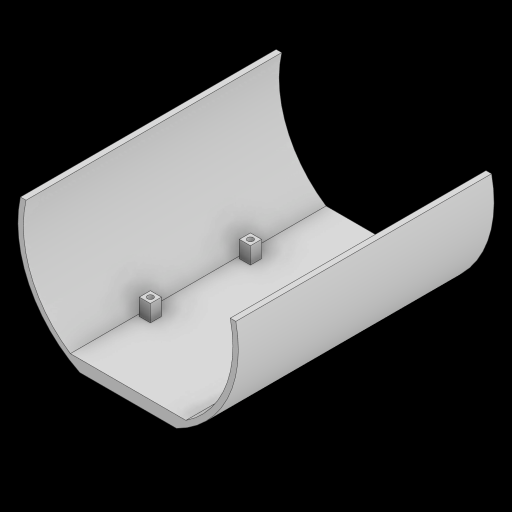
# Autodesk Inventor part: BackInsertV1
Saved by Autodesk Inventor 2024 (Build 280153000, 153)
## iProperties
Created: 2026-04-20
Part Number: BackInsertV1
Material: Generic
Document SubType Name: Modeling
Designer: Tanner
Density: 1 g/cm^3
Appearance: Default
Author: Tanner
## iProperties of the stored document BackInsertV1_3DPrint.ipt
Created: 2026-04-27
Part Number: BackInsertV1_3DPrint
Material: Generic
Document SubType Name: Modeling
Designer: Tanner
Density: 1 g/cm^3
Appearance: Default
Author: Tanner
Autodesk Inventor part; units mm, degrees
ref_plane "YZ Plane" through (0, 0, 0) normal (1, 0, 0) x (0, 1, 0)
ref_plane "XZ Plane" through (0, 0, 0) normal (0, 1, 0) x (-1, 0, 0)
ref_plane "XY Plane" through (0, 0, 0) normal (0, 0, 1) x (1, 0, 0)
sketch "Sketch1" plane through (0, 0, 0) normal (0, 0, 1) x (1, 0, 0)
  arc A0 (-96.8589, 55) -> (-43.4971, -55) centre (0, 34.0439) ccw projected
  line L0 (-43.4971, -55) -> (43.4971, -55) projected
  arc A1 (43.4971, -55) -> (96.8589, 55) centre (0, 34.0439) ccw projected
  line L1 (96.8589, 55) -> (91.8589, 55) projected
  arc A2 (51.9882, -44.5338) -> (91.8589, 55) centre (0, 34.0439) ccw projected
  arc A3 (-91.8589, 55) -> (-51.9882, -44.5338) centre (0, 34.0439) ccw projected
  line L2 (-91.8589, 55) -> (-96.8589, 55) projected
  line L3 (51.9882, -44.5338) -> (-51.9882, -44.5338) projected
  point P0 (0, 0)
extrude "Extrusion1" add sketch "Sketch1" along normal blind 230
sketch "Sketch2" plane through (-43.4971, -44.5338, 0) normal (0, 1, 0) x (1, 0, 0)
  circle A0 centre (-1.5029, -75) radius 1.6 construction
  circle A1 centre (-1.5029, -165) radius 1.6 construction
  circle A2 centre (88.4971, -75) radius 1.6 construction
  circle A3 centre (88.4971, -165) radius 1.6 construction
  line L0 (-6.5029, -70) -> (-6.5029, -170) construction
  line L1 (-6.5029, -170) -> (93.4971, -170) construction
  line L2 (93.4971, -170) -> (93.4971, -70) construction
  line L3 (93.4971, -70) -> (-6.5029, -70) construction
  line L4 (86.9943, 0) -> (0, 0) construction
  line L5 (0, 0) -> (0, -230) construction
  line L6 (86.9943, -230) -> (0, -230) construction
  line L7 (86.9943, 0) -> (86.9943, -230) construction
  line L8 (-6.5029, -80) -> (3.4971, -80)
  line L9 (3.4971, -80) -> (3.4971, -70)
  line L10 (3.4971, -70) -> (-6.5029, -70)
  line L11 (-6.5029, -70) -> (-6.5029, -80)
  line L12 (-6.5029, -80) -> (3.4971, -70) construction
  line L13 (3.4971, -80) -> (-6.5029, -70) construction
  line L14 (83.4971, -80) -> (93.4971, -80)
  line L15 (93.4971, -80) -> (93.4971, -70)
  line L16 (93.4971, -70) -> (83.4971, -70)
  line L17 (83.4971, -70) -> (83.4971, -80)
  line L18 (83.4971, -80) -> (93.4971, -70) construction
  line L19 (93.4971, -80) -> (83.4971, -70) construction
  line L20 (3.4971, -170) -> (-6.5029, -170)
  line L21 (-6.5029, -170) -> (-6.5029, -160)
  line L22 (-6.5029, -160) -> (3.4971, -160)
  line L23 (3.4971, -160) -> (3.4971, -170)
  line L24 (3.4971, -170) -> (-6.5029, -160) construction
  line L25 (-6.5029, -170) -> (3.4971, -160) construction
  line L26 (83.4971, -170) -> (93.4971, -170)
  line L27 (93.4971, -170) -> (93.4971, -160)
  line L28 (93.4971, -160) -> (83.4971, -160)
  line L29 (83.4971, -160) -> (83.4971, -170)
  line L30 (83.4971, -170) -> (93.4971, -160) construction
  line L31 (93.4971, -170) -> (83.4971, -160) construction
  point P0 (43.4971, 0)
  dimension "d2" = 10
  dimension "d3" = 10
  dimension "d4" = 10
  dimension "d5" = 10
  dimension "d6" = 10
  dimension "d7" = 10
  dimension "d8" = 10
  dimension "d9" = 10
  constraints: 48 end point, 8 midpoint, 8 parallel, 4 horizontal, 4 perpendicular
  measures "d2" distance of L10.end L9.end
  measures "d3" distance of L9.end L8.end
  measures "d4" distance of L16.end L15.end
  measures "d5" distance of L15.end L14.end
  measures "d6" distance of L21.end L22.end
  measures "d7" distance of L20.end L21.end
  measures "d8" distance of L28.end L27.end
  measures "d9" distance of L27.end L26.end
extrude "Extrusion2" add sketch "Sketch2" along normal blind 15
sketch "Sketch3" plane through (-43.4971, -29.5338, 0) normal (0, 1, 0) x (1, 0, 0)
  circle A0 centre (-1.5029, -75) radius 1.6 construction
  circle A1 centre (-1.5029, -165) radius 1.6 construction
  circle A2 centre (88.4971, -75) radius 1.6 construction
  circle A3 centre (88.4971, -165) radius 1.6 construction
  line L0 (-6.5029, -70) -> (-6.5029, -170) construction
  line L1 (-6.5029, -170) -> (93.4971, -170) construction
  line L2 (93.4971, -170) -> (93.4971, -70) construction
  line L3 (93.4971, -70) -> (-6.5029, -70) construction
  circle A4 centre (-1.5029, -75) radius 2.665
  circle A5 centre (88.4971, -75) radius 2.665
  circle A6 centre (88.4971, -165) radius 2.665
  circle A7 centre (-1.5029, -165) radius 2.665
  point P0 (43.4971, 0)
  dimension "d12" = 5.33
  dimension "d13" = 5.33
  dimension "d14" = 5.33
  dimension "d15" = 5.33
  constraints: 4 centre point, 4 coincident
  measures "d12" diameter of A4
  measures "d13" diameter of A5
  measures "d14" diameter of A6
  measures "d15" diameter of A7
extrude "Extrusion3" cut sketch "Sketch3" against normal blind 11.5
sketch "Sketch4" plane through (0, 0, 0) normal (0, 0, -1) x (-1, 0, 0)
  arc A0 (43.4971, -55) -> (96.8589, 55) centre (0, 34.0439) ccw construction
  line L0 (43.4971, -55) -> (-43.4971, -55) construction
  arc A1 (-96.8589, 55) -> (-43.4971, -55) centre (0, 34.0439) ccw construction
  line L1 (-96.8589, 55) -> (-91.8589, 55) construction
  arc A2 (-91.8589, 55) -> (-51.9882, -44.5338) centre (0, 34.0439) ccw construction
  line L2 (-51.9882, -44.5338) -> (51.9882, -44.5338) construction
  arc A3 (51.9882, -44.5338) -> (91.8589, 55) centre (0, 34.0439) ccw construction
  line L3 (91.8589, 55) -> (96.8589, 55) construction
  arc A4 (43.4971, -55) -> (96.8589, 55) centre (0, 34.0439) ccw construction
  line L4 (43.4971, -55) -> (-43.4971, -55) construction
  arc A5 (-96.8589, 55) -> (-43.4971, -55) centre (0, 34.0439) ccw construction
  line L5 (-96.8589, 55) -> (-91.8589, 55) construction
  arc A6 (-91.8589, 55) -> (-51.9882, -44.5338) centre (0, 34.0439) ccw construction
  arc A7 (51.9882, -44.5338) -> (91.8589, 55) centre (0, 34.0439) ccw construction
  line L6 (91.8589, 55) -> (96.8589, 55) construction
  line L7 (-51.9882, -44.5338) -> (51.9882, -44.5338)
  line L8 (47.665, -29.5338) -> (47.665, -41.0338) projected
  line L9 (-43.4971, -49.5338) -> (43.4971, -49.5338)
  arc A8 (-51.9882, -44.5338) -> (-43.4971, -49.5338) centre (0, 34.0439) ccw
  arc A9 (43.4971, -49.5338) -> (51.9882, -44.5338) centre (0, 34.0439) ccw
  arc A10 (43.4971, -49.5338) -> (91.8589, 55) centre (0, 34.0439) ccw projected
  line L10 (-51.9882, -44.5338) -> (51.9882, -44.5338) projected
  point P0 (0, 0)
  constraints: 4 end point, 4 point on circle, 2 centre point, 2 concentric, 1 perpendicular
extrude "Extrusion4" add sketch "Sketch4" against normal blind 30
body "Solid1"
